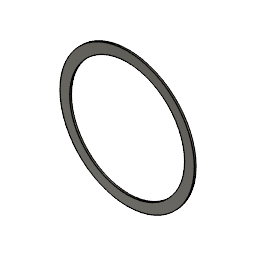
THE FINAL ASSEMBLY OF  LASER CUTTING (Autodesk Fusion 360 archive; units mm, degrees)
design "first ring after centre"
part number: 2026-02-17-13-51-02-636
Autodesk Fusion 360 part; units mm, degrees
sketch "Sketch1" plane through (0, 0, 0) normal (0, 1, 0) x (1, 0, 0)
  circle A0 centre (0, 0) radius 70
  circle A1 centre (0, 0) radius 82.1
  dimension "d9" = 140
  dimension "d10" = 164.2
  constraint coincident A0.centre A1.centre
  constraint concentric A0 A1
  measures "d9" diameter of A0
  measures "d10" diameter of A1
extrude "Extrude1" add sketch "Sketch1" along normal blind 2

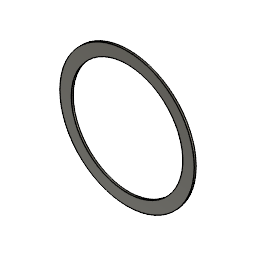
design "second ring after center"
part number: 2026-02-17-13-49-51-627
Autodesk Fusion 360 part; units mm, degrees
sketch "Sketch1" plane through (0, 0, 0) normal (0, 1, 0) x (1, 0, 0)
sketch "Sketch2" plane through (0, 0, 0) normal (0, 1, 0) x (1, 0, 0)
  circle A0 centre (0, 0) radius 60
  circle A1 centre (0, 0) radius 72.45
  dimension "d18" = 120
  dimension "d19" = 144.9
  constraint coincident A0.centre A1.centre
  measures "d18" diameter of A0
  measures "d19" diameter of A1
extrude "Extrude3" add sketch "Sketch2" along normal blind 2

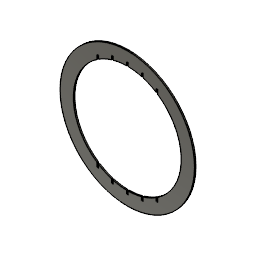
design "lastring"
part number: 2026-02-18-20-44-55-759
Autodesk Fusion 360 part; units mm, degrees
sketch "Sketch1" plane through (0, 0, 0) normal (0, 1, 0) x (1, 0, 0)
  line L0 (-0.9547, -79.9943) -> (-1.0144, -84.9943)
  line L1 (-1.0144, -84.9943) -> (0.9855, -85.0182)
  line L2 (-21.2219, -77.1338) -> (-21.2816, -82.1335)
  line L3 (-21.2816, -82.1335) -> (-23.2814, -82.1096)
  line L4 (-23.2814, -82.1096) -> (-23.2152, -76.5575)
  line L5 (-42.9575, -67.4881) -> (-42.9575, -72.4881)
  line L6 (-42.9575, -72.4881) -> (-44.9575, -72.4881)
  line L7 (-44.9575, -72.4881) -> (-44.9575, -66.1727)
  arc A0 (-42.9575, -67.4881) -> (-23.2152, -76.5575) centre (0, 0) ccw
  arc A1 (-21.2219, -77.1338) -> (-0.9547, -79.9943) centre (0, 0) ccw
  line L8 (-0.9547, 79.9943) -> (-0.9547, 84.9943)
  line L9 (-0.9547, 84.9943) -> (-0.0144, 84.9943)
  line L10 (-21.2219, 77.1338) -> (-21.2219, 82.1338)
  line L11 (-21.2219, 82.1338) -> (-23.2219, 82.1338)
  line L12 (-23.2219, 82.1338) -> (-23.2219, 76.5555)
  line L13 (-42.9575, 67.4881) -> (-42.9575, 72.4881)
  line L14 (-42.9575, 72.4881) -> (-44.9575, 72.4881)
  line L15 (-44.9575, 72.4881) -> (-44.9575, 66.1727)
  arc A2 (-44.9575, 66.1727) -> (-44.9575, -66.1727) centre (0, 0) ccw
  arc A3 (-23.2219, 76.5555) -> (-42.9575, 67.4881) centre (0, 0) ccw
  arc A4 (-0.9547, 79.9943) -> (-21.2219, 77.1338) centre (0, 0) ccw
  line L16 (42.9286, 72.4881) -> (44.9286, 72.4881)
  line L17 (21.2527, -82.1335) -> (23.2525, -82.1096)
  arc A5 (21.193, 77.1338) -> (0.9258, 79.9943) centre (-0.0289, 0) ccw
  line L18 (0.9258, -79.9943) -> (0.9855, -84.9943)
  line L19 (23.2525, -82.1096) -> (23.1863, -76.5575)
  arc A6 (0.9258, -79.9943) -> (21.193, -77.1338) centre (-0.0289, 0) ccw
  line L20 (21.193, -77.1338) -> (21.2527, -82.1335)
  arc A7 (44.9286, -66.1727) -> (44.9286, 66.1727) centre (-0.0289, 0) ccw
  line L21 (42.9286, 67.4881) -> (42.9286, 72.4881)
  line L22 (21.193, 77.1338) -> (21.193, 82.1338)
  line L23 (21.193, 82.1338) -> (23.193, 82.1338)
  line L24 (42.9286, -72.4881) -> (44.9286, -72.4881)
  line L25 (44.9286, -72.4881) -> (44.9286, -66.1727)
  arc A8 (23.1863, -76.5575) -> (42.9286, -67.4881) centre (-0.0289, 0) ccw
  line L26 (23.193, 82.1338) -> (23.193, 76.5555)
  line L27 (42.9286, -67.4881) -> (42.9286, -72.4881)
  line L28 (0.9258, 84.9943) -> (-0.0144, 84.9943)
  line L29 (0.9258, 79.9943) -> (0.9258, 84.9943)
  line L30 (44.9286, 72.4881) -> (44.9286, 66.1727)
  arc A9 (42.9286, 67.4881) -> (23.193, 76.5555) centre (-0.0289, 0) ccw
  line L31 (0.9855, -84.9943) -> (-1.0144, -85.0182)
  circle A10 centre (-0.0289, 0) radius 100
  point P0 (-0.0289, 0)
  dimension "d2" = 2
  dimension "d3" = 5
  dimension "d6" = 2
  dimension "d20" = 200
  constraint coincident A0.centre A1.centre
  constraint coincident A0.centre L0
  constraint perpendicular L0 L1
  constraint perpendicular L2 L3
  constraint perpendicular L3 L4
  constraint vertical L5
  constraint perpendicular L5 L6
  constraint perpendicular L6 L7
  constraint concentric A0 A1
  constraint perpendicular L8 L9
  constraint perpendicular L10 L11
  constraint perpendicular L11 L12
  constraint perpendicular L13 L14
  constraint perpendicular L14 L15
  constraint concentric A2 A3
  constraint concentric A3 A4
  constraint concentric A8 A10
  measures "d2" distance of L0.end L1.end
  measures "d3" vertical distance of L0.start L0.end
  measures "d6" distance of L2.end L3.end
  measures "d20" diameter of A10
extrude "Extrude3" add sketch "Sketch1" along normal blind 2
extrude "Extrude2" [suppressed]

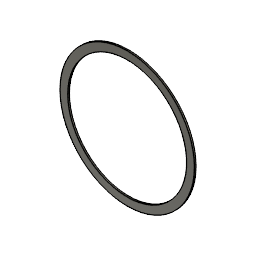
design "centre ring"
part number: 2026-02-17-14-00-17-370
Autodesk Fusion 360 part; units mm, degrees
sketch "Sketch3" plane through (0, 0, 0) normal (0, 1, 0) x (1, 0, 0)
  circle A0 centre (0, 0) radius 85
  circle A1 centre (0, 0) radius 75
  dimension "d10" = 170
  dimension "d11" = 150
  constraint coincident A0.centre A1.centre
  constraint concentric A0 A1
  measures "d10" diameter of A0
  measures "d11" diameter of A1
extrude "Extrude3" add sketch "Sketch3" along normal blind 2
